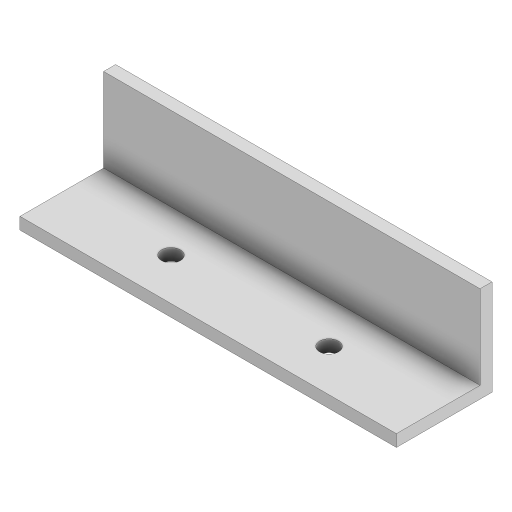
# Autodesk Inventor part: SOPORTE LATERAL DE GUIA CILINDRICA
Saved by Autodesk Inventor 2024 (Build 280153000, 153)
## iProperties
Created: 2024-06-22
Part Number: SOPORTE LATERAL DE GUIA CILINDRICA
Material: Generic
Document SubType Name: Modeling
Designer: Jhuliams
Density: 1 g/cm^3
Appearance: Default
Author: Jhuliams
Autodesk Inventor part; units mm, degrees
ref_plane "YZ Plane" through (0, 0, 0) normal (1, 0, 0) x (0, 1, 0)
ref_plane "XZ Plane" through (0, 0, 0) normal (0, 1, 0) x (-1, 0, 0)
ref_plane "XY Plane" through (0, 0, 0) normal (0, 0, 1) x (1, 0, 0)
sketch "Sketch1" plane through (0, 0, 0) normal (1, 0, 0) x (0, 1, 0)
  line L0 (0, 0) -> (25.4, 0)
  line L1 (25.4, 0) -> (25.4, 3.175)
  line L2 (25.4, 3.175) -> (0, 3.175)
  line L3 (0, 3.175) -> (0, 0)
  line L4 (0, 0) -> (0, 25.4)
  line L5 (0, 25.4) -> (3.175, 25.4)
  line L6 (3.175, 25.4) -> (3.175, 3.175)
  point P0 (3.175, 3.175)
  dimension "d0" = 25.4
  dimension "d1" = 3.175
  dimension "d2" = 25.4
  dimension "d3" = 25.4
  dimension "d4" = 3.175
  dimension "d5" = 90
  constraints: 14 end point, 3 perpendicular, 1 horizontal, 1 vertical
  measures "d0" distance of L0.start L0.end
  measures "d1" distance of L0.end L1.end
  measures "d2" distance of L1.end L2.end
  measures "d3" distance of L0.start L4.end
  measures "d4" distance of L4.end L5.end
  measures "d5" angle of L4 L5
extrude "Extrusion1" add sketch "Sketch1" along normal blind 100
sketch "Sketch2" plane through (0, 3.175, 25.4) normal (0, 1, 0) x (1, 0, 0)
  line L0 (0, 22.225) -> (0, 0) projected
  line L1 (0, 0) -> (100, 0) projected
  line L2 (100, 22.225) -> (100, 0) projected
  line L3 (0, 22.225) -> (100, 22.225) projected
  line L4 (0, 0) -> (100, 22.225)
  line L5 (0, 22.225) -> (100, 0)
  line L6 (50, 11.1125) -> (29, 11.1125)
  line L7 (29, 11.1125) -> (71, 11.1125)
  circle A0 centre (29, 11.1125) radius 2.5
  circle A1 centre (71, 11.1125) radius 2.5
  point P0 (0, 25.4)
  dimension "d8" = 21
  dimension "d9" = 42
  dimension "d10" = 5
  dimension "d11" = 5
  constraints: 8 end point, 2 centre point, 2 coincident, 1 horizontal, 1 midpoint, 1 point on line
  measures "d8" distance of L6.start L6.end
  measures "d9" distance of L6.end L7.end
  measures "d10" diameter of A0
  measures "d11" diameter of A1
extrude "Extrusion2" cut sketch "Sketch2" against normal blind 10 contours A0 | A1
body "Solid1"
